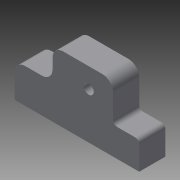
# Autodesk Inventor part: other side roller axle holder
Saved by Autodesk Inventor 2015 (Build 190159000, 159)
## iProperties
Created: 2014-09-20
Part Number: other side roller axle holder
Material: Generic
Document SubType Name: Modeling
Designer: jesse
Density: 1 g/cm^3
Appearance: Default
Author: jesse
Autodesk Inventor part; units mm, degrees
ref_plane "YZ Plane" through (0, 0, 0) normal (1, 0, 0) x (0, 1, 0)
ref_plane "XZ Plane" through (0, 0, 0) normal (0, 1, 0) x (-1, 0, 0)
ref_plane "XY Plane" through (0, 0, 0) normal (0, 0, 1) x (1, 0, 0)
ref_plane "FRONT" through (0, 0, 0) normal (0, 0, 1) x (1, 0, 0)
ref_plane "TOP" through (0, 0, 0) normal (0, 1, 0) x (-1, 0, 0)
ref_plane "RIGHT" through (0, 0, 0) normal (1, 0, 0) x (0, 1, 0)
ref_plane "Work Plane6" through (36, -22.5, -6.35) normal (0, 0, -1) x (-1, 0, 0)
sketch "Sketch1" plane through (36, -22.5, -6.35) normal (0, 0, -1) x (-1, 0, 0)
  line L0 (72, 0) -> (0, 0) projected
  line L1 (72, 0) -> (24.2203, 0)
  line L2 (72, 0) -> (0, 0) projected
  line L3 (24.2203, 0) -> (24.2203, 32.1053)
  line L4 (24.2203, 32.1053) -> (53.5869, 32.1053)
  line L5 (53.5869, 32.1053) -> (53.5869, 16.7597)
  arc A0 (54.4391, 24) -> (54.4391, 21) centre (36, 22.5) ccw projected
  line L6 (53.5869, 16.7597) -> (72, 16.7597)
  line L7 (72, 16.7597) -> (72, 0)
  constraints: 12 end point, 3 perpendicular, 1 horizontal, 1 point on circle, 1 point on line, 1 vertical
extrude "Extrusion1" add sketch "Sketch1" along normal blind 12.7 contours L0 L3 A0 L6 L7 | L3 L4 A0 L5 | L4 L5 A0
ref_plane "Work Plane5" through (36, -22.5, -19.05) normal (0, 0, -1) x (-1, 0, 0)
sketch "Sketch2" plane through (36, -22.5, -19.05) normal (0, 0, -1) x (-1, 0, 0)
  circle A0 centre (36, 22.5) radius 2.3812
  dimension "d2" = 4.7625
  constraints: 1 centre point, 1 coincident
  measures "d2" diameter of A0
extrude "Extrusion2" cut sketch "Sketch2" against normal through all
fillet "Fillet1" radius 5.175 1 edges at (-17.5869, -5.7403, -12.7)
fillet "Fillet2" radius 5.175 3 edges at (-17.5869, 9.6053, -12.7) (-36, -5.7403, -12.7) (11.7797, 9.6053, -12.7)
sketch "Sketch3" plane through (11.7797, -22.5, -6.35) normal (1, 0, 0) x (0, 0, -1)
  line L0 (0, 26.9303) -> (0, 0) projected
  line L1 (0, 13.4651) -> (12.7, 13.4651)
  line L2 (12.7, 13.4651) -> (12.7, 0)
  line L3 (12.7, 0) -> (0, 0)
  line L4 (0, 0) -> (0, 13.4651)
  point P0 (-6.35, 22.5)
  constraints: 8 end point, 2 parallel, 1 horizontal, 1 midpoint, 1 perpendicular
extrude "Extrusion3" add sketch "Sketch3" along normal blind 12.7
fillet "Fillet3" radius 2 2 edges at (11.7797, -9.0349, -12.7) (24.4797, -9.0349, -12.7)
